Autodesk Fusion 360 part; units mm, degrees
(part 6 of 6)
  line L47 (66.5472, -12.2089) -> (65.9278, -12.0953)
  arc A95 (64.3117, -9.8261) -> (65.9278, -12.0953) centre (66.2887, -10.1281) ccw
  circle A96 centre (0, 0) radius 2.45
  ellipse E0 centre (-99.2333, 63.826) end of major axis (-99.2333, 23.826) minor radius 30
  circle A97 centre (-96.6709, 10.0468) radius 6
  circle A98 centre (-99.1793, -9.1662) radius 3.25
  circle A99 centre (-93.7424, -33.2888) radius 10
  circle A100 centre (-93.7424, -33.2888) radius 6
  circle A101 centre (-93.7424, -33.2888) radius 6
  circle A102 centre (-93.7424, -33.2888) radius 10
  circle A103 centre (-74.9782, -57.1169) radius 6
  circle A104 centre (-74.9782, -57.1169) radius 10
  circle A105 centre (0, 0) radius 6
  circle A106 centre (0, 0) radius 10
  circle A107 centre (-99.2333, 63.826) radius 6
  circle A108 centre (-99.2333, 63.826) radius 10
named bodies: "Spur Gear (24 teeth)", "Cap", "Spacer 1", "Spacer 2", "Back Cap", "Cam"
